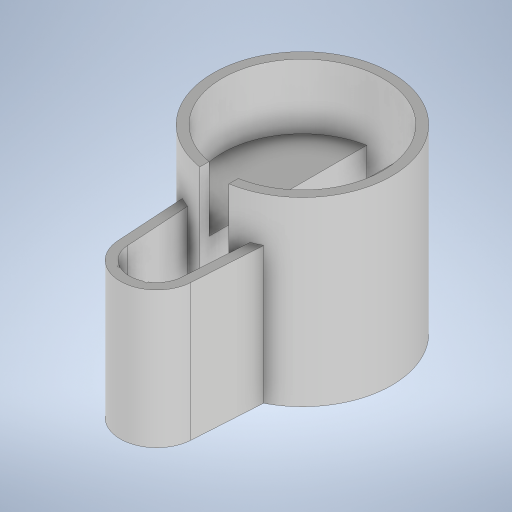
# Autodesk Inventor part: Servo Adapter 4
Saved by Autodesk Inventor 2024 (Build 280153000, 153)
## iProperties
Created: 2023-02-08
Part Number: Servo Adapter 4
Material: Generic
Document SubType Name: Modeling
Designer: tommy
Density: 1 g/cm^3
Appearance: Default
Author: tommy
Autodesk Inventor part; units mm, degrees
ref_plane "YZ Plane" through (0, 0, 0) normal (1, 0, 0) x (0, 1, 0)
ref_plane "XZ Plane" through (0, 0, 0) normal (0, 1, 0) x (-1, 0, 0)
ref_plane "XY Plane" through (0, 0, 0) normal (0, 0, 1) x (1, 0, 0)
sketch "Valve Handle" plane through (0, 0, 0) normal (0, 0, 1) x (1, 0, 0)
  line L0 (-2.032, 23.7871) -> (2.032, 23.7871)
  line L1 (-2.032, -23.7871) -> (2.032, -23.7871)
  line L2 (-2.032, 23.7871) -> (-2.032, -23.7871)
  line L3 (2.032, 23.7871) -> (2.032, -23.7871)
  line L4 (0, 11.176) -> (0, -22.606)
  line L5 (0, 11.176) -> (0, -22.606)
  point P0 (0, -1.7145)
  point P1 (0, 0)
  dimension "d146" = 33.782
  dimension "d167" = 11.176
  dimension "d168" = 22.606
  measures "d146" distance of L4.start L4.end
  measures "d167" distance of L4.start point (0, 0)
  measures "d168" distance of L4.end point (0, 0)
sketch "Valve Casing" plane through (0, 0, 0) normal (0, 0, 1) x (1, 0, 0)
  circle A0 centre (0, 0) radius 8.636
  circle A1 centre (0, 0) radius 11.176
  circle A2 centre (0, 0) radius 12.446
  dimension "d149" = 24.892
  measures "d149" diameter of A2
sketch "Servo Arm Socket" plane through (0, 0, 0) normal (0, 0, 1) x (1, 0, 0)
  arc A0 (4.8166, -0.3016) -> (-4.8166, -0.3016) centre (0, 0) ccw
  line L0 (0, 0) -> (0, -20.32)
  arc A1 (-3.549, -20.5423) -> (3.549, -20.5423) centre (0, -20.32) ccw
  line L1 (-3.549, -20.5423) -> (-4.8166, -0.3016)
  line L2 (4.8166, -0.3016) -> (3.549, -20.5423)
  line L3 (-5.0701, -0.3175) -> (-3.8026, -20.5581)
  arc A2 (-3.8026, -20.5581) -> (3.8026, -20.5581) centre (0, -20.32) ccw
  line L4 (3.8026, -20.5581) -> (5.0701, -0.3175)
  arc A3 (5.0701, -0.3175) -> (-5.0701, -0.3175) centre (0, 0) ccw
  line L5 (-5.0701, -20.6375) -> (-6.3376, -0.3969)
  arc A4 (6.3376, -0.3969) -> (-6.3376, -0.3969) centre (0, 0) ccw
  line L6 (6.3376, -0.3969) -> (5.0701, -20.6375)
  arc A5 (-5.0701, -20.6375) -> (5.0701, -20.6375) centre (0, -20.32) ccw
  dimension "d162" = 9.652
  dimension "d163" = 20.32
  dimension "d164" = 7.112
  dimension "d165" = 0.254
  dimension "d166" = 1.27
  measures "d162" diameter of A0
  measures "d163" distance of L0.start L0.end
  measures "d164" diameter of A1
  measures "d165" distance between parallel lines of L1 L3
  measures "d166" distance between parallel lines of L3 L5
sketch "Sketch10" plane through (0, 0, 0) normal (0, 1, 0) x (-1, 0, 0)
  line L0 (0, -14.097) -> (0, 0)
  line L1 (0, 23.7871) -> (0, -23.7871) construction
  line L2 (-2.032, 23.7871) -> (2.032, 23.7871)
  line L3 (-2.032, -23.7871) -> (2.032, -23.7871)
  line L4 (-2.032, 23.7871) -> (-2.032, -23.7871)
  line L5 (2.032, 23.7871) -> (2.032, -23.7871)
  line L6 (0, 11.176) -> (0, -22.606)
  line L7 (0, 11.176) -> (0, -22.606)
  circle A0 centre (0, 0) radius 8.636
  circle A1 centre (0, 0) radius 11.176
  circle A2 centre (0, 0) radius 12.446
  arc A3 (4.8166, -0.3016) -> (-4.8166, -0.3016) centre (0, 0) ccw
  line L8 (0, 0) -> (0, -20.32)
  arc A4 (-3.549, -20.5423) -> (3.549, -20.5423) centre (0, -20.32) ccw
  line L9 (-3.549, -20.5423) -> (-4.8166, -0.3016)
  line L10 (4.8166, -0.3016) -> (3.549, -20.5423)
  line L11 (-5.0701, -0.3175) -> (-3.8026, -20.5581)
  arc A5 (-3.8026, -20.5581) -> (3.8026, -20.5581) centre (0, -20.32) ccw
  line L12 (3.8026, -20.5581) -> (5.0701, -0.3175)
  arc A6 (5.0701, -0.3175) -> (-5.0701, -0.3175) centre (0, 0) ccw
  line L13 (-5.0701, -20.6375) -> (-6.3376, -0.3969)
  arc A7 (6.3376, -0.3969) -> (-6.3376, -0.3969) centre (0, 0) ccw
  line L14 (6.3376, -0.3969) -> (5.0701, -20.6375)
  arc A8 (-5.0701, -20.6375) -> (5.0701, -20.6375) centre (0, -20.32) ccw
  point P0 (2.032, -10.9897)
  point P1 (2.032, -12.279)
  point P2 (-2.032, -12.279)
  point P3 (-2.032, -10.9897)
  point P4 (-2.032, 10.9897)
  point P5 (2.032, 10.9897)
  point P6 (-6.1771, -11.0965)
  point P7 (6.1771, -11.0965)
  point P8 (6.4453, -9.1302)
  point P9 (7.0009, -5.0565)
  point P10 (2.032, 8.3935)
  point P11 (-2.032, 8.3935)
  point P12 (-7.0009, -5.0565)
  point P13 (6.1771, -11.0965)
  point P14 (-6.1771, -11.0965)
  point P15 (2.032, 7.3441)
  point P16 (-7.0009, -5.0565)
  point P17 (7.0009, -5.0565)
  point P18 (6.4453, -9.1302)
  point P19 (2.032, -19.4386)
  point P20 (-6.4453, -9.1302)
  point P21 (2.032, -8.3935)
  point P22 (-2.032, 7.3441)
  point P23 (-2.032, -19.4386)
  point P24 (-2.032, -8.3935)
  point P25 (-5.6686, -11.0802)
  point P26 (5.6686, -11.0802)
  point P27 (5.9718, -6.2385)
  point P28 (-5.9718, -6.2385)
  point P29 (5.7628, -9.5757)
  point P30 (-5.7628, -9.5757)
  point P31 (4.3599, -11.6574)
  point P32 (2.032, -23.5429)
  point P33 (1.5797, -23.7871)
  point P34 (-1.5797, -23.7871)
  point P35 (-2.032, -23.5429)
  point P36 (-4.3599, -11.6574)
  constraints: 5 vertical, 4 end point, 4 other
extrude "Extrusion21" add sketch "Sketch10" against normal blind 17.145 contours A2 L9 A1 L4 | L5 A1 L10 A2 | A2 L11 A1 L9 | L10 A1 L12 A2 | A2 L13 A1 L11 | L12 A1 L14 A2 | A2 L4 A1 L13 | L14 A1 L5 A2 | A2 L5 A1 L4
extrude "Extrusion22" add sketch "Sketch10" against normal blind 8.128 contours A1 L9 A0 L4 | L5 A0 L10 A1 | A0 L9 A3 L4 | L5 A3 L10 A0 | A1 L11 A0 L9 | L10 A0 L12 A1 | A3 L9 A0 L11 A6 L4 | L5 A6 L12 A0 L10 A3 | A1 L13 A0 L11 | L12 A0 L14 A1 | A6 L11 A0 L13 A7 L4 | L5 A7 L14 A0 L12 A6 | A1 L4 A0 L13 | L14 A0 L5 A1 | A7 L13 A0 L4 | L5 A0 L14 A7
extrude "Extrusion25" add sketch "Sketch10" along normal blind 8.128 contours A5 L3 L4 | L4 L3 A5 L5 L12 A2 L14 A8 L13 L11 | A2 L13 A1 L11 | L5 L3 A5 | L12 A1 L14 A2 | A1 L13 A0 L11 | L12 A0 L14 A1 | A2 L4 A1 L13 | L14 A1 L5 A2 | A6 L4 A7 L6 | L6 A7 L5 A6 | A6 L11 A0 L13 A7 L4 | L5 A7 L14 A0 L12 A6 | A2 L5 A1 L4 | A7 L4 A0 L6 | L6 A0 L5 A7 | A7 L13 A0 L4 | L5 A0 L14 A7 | A1 L6 A0 L4 | L6 A1 L5 A0
sketch "Sketch11" plane through (0, 0, 0) normal (0, 0, 1) x (1, 0, 0)
  point P0 (0, 0)
extrude "Extrusion27" add sketch "Sketch10" against normal blind 10.922 contours L4 L3 A5 L5 L12 A2 L14 A8 L13 L11
body "Solid1"
